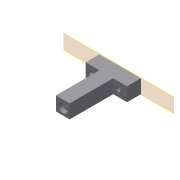
# Autodesk Inventor part: 00_3rdleg
Saved by Autodesk Inventor 2019.4 (Build 234330000, 330)
## iProperties
Created: 2020-11-15
Part Number: 00_3rdleg
Material: Generic
Document SubType Name: Modeling
Designer: diederichbenedict
Density: 1 g/cm^3
Appearance: Default
Author: diederichbenedict
Autodesk Inventor part; units mm, degrees
ref_plane "YZ Plane" through (0, 0, 0) normal (1, 0, 0) x (0, 1, 0)
ref_plane "XZ Plane" through (0, 0, 0) normal (0, 1, 0) x (-1, 0, 0)
ref_plane "XY Plane" through (0, 0, 0) normal (0, 0, 1) x (1, 0, 0)
ref_plane "Work Plane1" through (0, 0, 0) normal (0, 0, 1) x (1, 0, 0)
sketch "Sketch1" plane through (0, 0, 0) normal (0, 0, 1) x (1, 0, 0)
  circle A0 centre (45.9084, 5) radius 1.45 projected
  circle A1 centre (25.9084, 5) radius 1.45 projected
  line L0 (-21.0053, 0) -> (95.5084, 0) projected
  line L1 (95.5084, 10) -> (-17.0053, 10) projected
  line L2 (22.2515, 0) -> (52.2515, 0)
  line L3 (52.2515, 0) -> (52.2515, 10)
  line L4 (52.2515, 10) -> (22.2515, 10)
  line L5 (22.2515, 10) -> (22.2515, 0)
  line L6 (22.2515, 0) -> (52.2515, 10) construction
  line L7 (52.2515, 0) -> (22.2515, 10) construction
  circle A2 centre (45.9084, 5) radius 1.6
  circle A3 centre (25.9084, 5) radius 1.6
  point P0 (0, 0)
  point P1 (37.2515, 5)
  dimension "d0" = 30
  dimension "d1" = 3.2
  dimension "d2" = 3.2
  constraints: 12 end point, 2 centre point, 2 coincident, 2 midpoint, 2 parallel, 1 horizontal, 1 perpendicular, 1 point on line
  measures "d0" distance of L4.end L3.end
  measures "d1" diameter of A2
  measures "d2" diameter of A3
extrude "Extrusion1" add sketch "Sketch1" along normal blind 10 contours L5 L1 L3 L0
sketch "Sketch2" plane through (0, 0, 10) normal (0, 0, 1) x (1, 0, 0)
  line L0 (95.5084, 10) -> (-17.0053, 10) projected
  circle A0 centre (-15.5458, 215.5) radius 2.15 projected
  circle A1 centre (-15.5458, 5) radius 2.15 projected
  circle A2 centre (88.9625, 5) radius 2.15 projected
  circle A3 centre (88.9625, 215.5) radius 2.15 projected
  circle A4 centre (-6.0916, 148.2) radius 1.45 projected
  circle A5 centre (77.9084, 141.8) radius 1.45 projected
  circle A6 centre (71.5084, 15.8) radius 1.45 projected
  circle A7 centre (-6.0916, 15.8) radius 1.45 projected
  circle A8 centre (-12.2916, 22) radius 1.45 projected
  circle A9 centre (77.7084, 22) radius 1.45 projected
  circle A10 centre (71.5084, 148.2) radius 1.45 projected
  circle A11 centre (-12.2916, 143.3875) radius 1.45 projected
  arc A12 (-3.9916, 144.2) -> (-7.9916, 140.2) centre (-3.9916, 140.2) ccw projected
  line L1 (-3.9916, 144.2) -> (69.4084, 144.2) projected
  arc A13 (73.4084, 140.2) -> (69.4084, 144.2) centre (69.4084, 140.2) ccw projected
  line L2 (73.4084, 140.2) -> (73.4084, 24.1) projected
  arc A14 (69.4084, 20.1) -> (73.4084, 24.1) centre (69.4084, 24.1) ccw projected
  line L3 (69.4084, 20.1) -> (-3.9916, 20.1) projected
  arc A15 (-7.9916, 24.1) -> (-3.9916, 20.1) centre (-3.9916, 24.1) ccw projected
  line L4 (-7.9916, 24.1) -> (-7.9916, 140.2) projected
  line L5 (-21.0053, 220.5) -> (-21.0053, 0) projected
  line L6 (-21.0053, 0) -> (95.5084, 0) projected
  line L7 (95.5084, 0) -> (95.5084, 220.5) projected
  line L8 (95.5084, 220.5) -> (-21.0053, 220.5) projected
  line L9 (52.2515, 0) -> (52.2515, 10) projected
  line L10 (22.2515, 10) -> (22.2515, 0) projected
  line L11 (-21.0053, 0) -> (95.5084, 0) projected
  line L12 (42.2515, 10) -> (32.2515, 10)
  line L13 (32.2515, 10) -> (32.2515, 0)
  line L14 (32.2515, 0) -> (42.2515, 0)
  line L15 (42.2515, 0) -> (42.2515, 10)
  line L16 (42.2515, 10) -> (32.2515, 0) construction
  line L17 (32.2515, 10) -> (42.2515, 0) construction
  point P0 (0, 0)
  point P1 (37.2515, 5)
  dimension "d5" = 10
  dimension "d6" = 10
  constraints: 12 end point, 2 midpoint, 2 parallel, 1 horizontal, 1 perpendicular
  measures "d5" distance of L14.end L13.end
  measures "d6" distance of L13.end L12.end
ref_plane "Work Plane2" through (-21.0916, 0, 41.5167) normal (0, 0, -1) x (0, 1, 0)
extrude "Extrusion2" add sketch "Sketch2" along normal up to surface (31.5167 mm away) contours L15 L6 L13 L0
sketch "Sketch3" plane through (32.2515, 10, 41.5167) normal (0, 0, 1) x (1, 0, 0)
  line L0 (10, -10) -> (10, 0) projected
  line L1 (0, 0) -> (0, -10) projected
  line L2 (-49.2569, 0) -> (63.2569, 0) projected
  line L3 (63.2569, -10) -> (-53.3431, -10) projected
  circle A0 centre (-47.7973, -5) radius 3.5 projected
  circle A1 centre (4.9569, -5) radius 3.5
  point P0 (-32.2515, -10)
  constraints: 1 centre point
hole "Hole1" at (37.2084, 5, 41.5167) direction (0, 0, -1) diameter 2.9 depth 25 tip angle 118 counterbore diameter 7 counterbore depth 3
body "Solid1"
